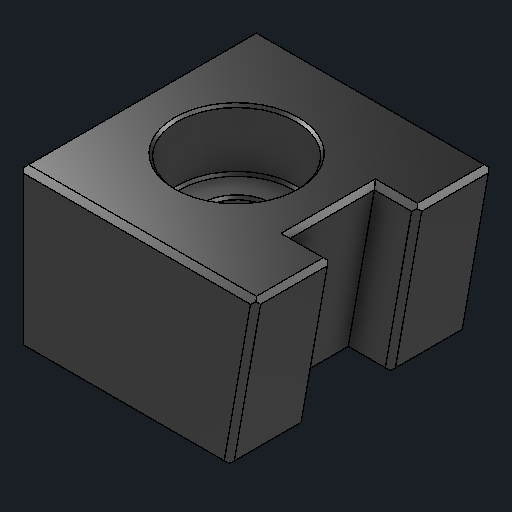
# Autodesk Inventor part: Fixture Jaw
Saved by Autodesk Inventor 2026.2 (Build 302298000, 298)
## iProperties
Created: 2026-05-18
Part Number: Fixture Jaw
Material: ABS Plastic
Document SubType Name: Modeling
Designer: JoshuaEah
Density: 1.06 g/cm^3
Appearance: Glossy - Black
Author: JoshuaEah
Autodesk Inventor part; units mm, degrees
ref_plane "YZ Plane" through (0, 0, 0) normal (1, 0, 0) x (0, 1, 0)
ref_plane "XZ Plane" through (0, 0, 0) normal (0, 1, 0) x (-1, 0, 0)
ref_plane "XY Plane" through (0, 0, 0) normal (0, 0, 1) x (1, 0, 0)
sketch "Sketch1" plane through (0, 0, 0) normal (0, 1, 0) x (-1, 0, 0)
  line L0 (0, 0) -> (-19.05, 0)
  line L1 (-19.05, 0) -> (-19.05, -19.05)
  line L2 (-19.05, -19.05) -> (0, -19.05)
  line L3 (0, -19.05) -> (0, 0)
  line L4 (0, -9.525) -> (-19.05, -9.525) construction
  line L5 (-15.875, -19.05) -> (-15.875, 0)
  line L6 (-15.875, -12.7) -> (-19.05, -12.7)
  line L7 (-15.875, -6.35) -> (-19.05, -6.35)
  circle A0 centre (-7.9375, -9.525) radius 3.175
  point P0 (-19.05, -6.35)
  point P1 (-15.875, -6.35)
  point P2 (-15.875, -12.7)
  point P3 (-19.05, -12.7)
  dimension "d0" = 19.05
  dimension "d1" = 19.05
  dimension "d2" = 3.175
  dimension "d3" = 6.35
  dimension "d15" = 6.35
  dimension "d16" = 7.9375
  constraints: 16 end point, 3 point on line, 2 midpoint, 2 parallel, 2 perpendicular, 2 symmetric about line, 1 centre point, 1 coincident, 1 horizontal
  measures "d0" distance of L2.end L1.end
  measures "d1" distance of L1.end L0.end
  measures "d2" distance between parallel lines of L1 L5
  measures "d3" diameter of L6 L4
  measures "d15" diameter of A0
  measures "d16" distance from line of L3 A0.centre
extrude "Extrusion1" add sketch "Sketch1" against normal blind 12.7 contours L3 L2 L5 L0 | L5 L7 L1 L0 | L5 L6 L1 L7 | L2 L1 L6 L5 | A0
hole "Hole1" at (7.9375, 0, -9.525) direction (0, -1, 0) diameter 5.1054 end through all counterbore diameter 9.525 counterbore depth 4.826 clearance for "Socket Head Cap Screw" size "#10" standard "Ansi Unified Screw Threads"
extrude "Extrusion2" cut sketch "Sketch1" against normal through all contours L5 L6 L1 L7
draft "FaceDraft2" angle 10 pull direction (0, -1, 0) faces at (19.05, -4.2333, -14.8167) (15.875, -4.2333, -10.5833) (19.05, -8.4667, -2.1167) fixed edges at (19.05, 0, -15.875) (15.875, 0, -9.525) (19.05, 0, -3.175)
thicken "Thicken1" operation cut thickness 0.2 both sides no extend neighbours yes toward (0, 0, 1) faces at (15.4404, -8.4667, -6.35) (14.3821, -8.4667, -8.4667) (17.2452, -4.2333, -12.7)
chamfer "Chamfer1" distance 0.4 angle 45 22 edges at (9.525, 0, 0) (0, 0, -9.525) (9.525, 0, -19.05) (19.05, 0, -15.975) (17.361, 0, -12.9) (15.6719, 0, -9.525) (17.361, 0, -6.15) (19.05, 0, -3.075) (8.4053, -12.7, 0) (16.8106, -12.7, -3.075) (15.1216, -12.7, -6.15) (13.4326, -12.7, -9.525) (15.1216, -12.7, -12.9) (16.8106, -12.7, -15.975) (8.4053, -12.7, -19.05) (0, -12.7, -9.525) (0, -6.35, 0) (0, -6.35, -19.05) (17.9303, -6.35, 0) (17.9303, -6.35, -6.15) (17.9303, -6.35, -12.9) (17.9303, -6.35, -19.05)
chamfer "Chamfer2" distance 0.2 angle 45 4 edges at (7.9375, 0, -14.2875) (7.9375, -4.826, -14.2875) (7.9375, -4.826, -12.0777) (7.9375, -12.7, -12.0777)
equation "\"d16\" = -0.5 * d2 + 0.5 * d0"
body "Solid1"
